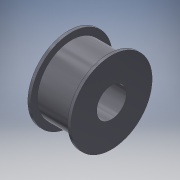
# Autodesk Inventor part: Solder Spool
Saved by Autodesk Inventor 2016 (Build 200138000, 138)
## iProperties
Created: 2017-09-04
Part Number: Solder Spool
Material: SAE 1020
Document SubType Name: Modeling
Designer: Zigunov
Stock Number: 0
Mass: 1729.01 g
Surface Area: 745.421 cm^2
Volume: 219.697 cm^3
Density: 7.87 g/cm^3
Appearance: Steel - Polished
Author: Zigunov
Autodesk Inventor part; units mm, degrees
ref_plane "YZ Plane" through (0, 0, 0) normal (1, 0, 0) x (0, 1, 0)
ref_plane "XZ Plane" through (0, 0, 0) normal (0, 1, 0) x (-1, 0, 0)
ref_plane "XY Plane" through (0, 0, 0) normal (0, 0, 1) x (1, 0, 0)
sketch "Sketch2" plane through (0, 0, 0) normal (0, 0, 1) x (1, 0, 0)
  line L0 (-14.5, 10) -> (14.5, 10)
  line L1 (14.5, 10) -> (14.5, 27.5)
  line L2 (14.5, 27.5) -> (12.5, 27.5)
  line L3 (12.5, 27.5) -> (12.5, 23)
  line L4 (12.5, 23) -> (-12.5, 23)
  line L5 (-12.5, 23) -> (-12.5, 27.5)
  line L6 (-12.5, 27.5) -> (-14.5, 27.5)
  line L7 (-14.5, 27.5) -> (-14.5, 10)
  line L8 (0, 0) -> (-7.6194, 0) construction
  line L9 (0, 0) -> (0, 10) construction
  dimension "d11" = 20
  dimension "d12" = 55
  dimension "d13" = 2
  dimension "d14" = 29
  dimension "d15" = 46
  constraints: 20 end point, 6 perpendicular, 2 horizontal, 2 point on line, 1 collinear, 1 midpoint, 1 vertical
  measures "d11" diameter of L0 L8
  measures "d12" diameter of L6 L8
  measures "d13" distance of L5.end L6.end
  measures "d14" distance between parallel lines of L1 L7
  measures "d15" diameter of L4 L8
revolve "Revolution1" add sketch "Sketch2" angle 360 about axis through (0, 0, 0) along (-1, 0, 0)
body "Solid2"
